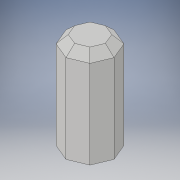
# Autodesk Inventor part: separator_battery
Saved by Autodesk Inventor 2019 (Build 230136000, 136)
## iProperties
Created: 2019-04-10
Part Number: separator_battery
Material: Generic
Document SubType Name: Modeling
Designer: jmc
Density: 1 g/cm^3
Appearance: Default
Author: jmc
Autodesk Inventor part; units mm, degrees
ref_plane "YZ Plane" through (0, 0, 0) normal (1, 0, 0) x (0, 1, 0)
ref_plane "XZ Plane" through (0, 0, 0) normal (0, 1, 0) x (-1, 0, 0)
ref_plane "XY Plane" through (0, 0, 0) normal (0, 0, 1) x (1, 0, 0)
sketch "Sketch1" plane through (0, 0, 0) normal (0, 1, 0) x (-1, 0, 0)
  circle A0 centre (0, 0) radius 1.5 construction
  line L0 (0, -1.5) -> (-1.0607, -1.0607)
  line L1 (-1.0607, -1.0607) -> (-1.5, 0)
  line L2 (-1.5, 0) -> (-1.0607, 1.0607)
  line L3 (-1.0607, 1.0607) -> (0, 1.5)
  line L4 (0, 1.5) -> (1.0607, 1.0607)
  line L5 (1.0607, 1.0607) -> (1.5, 0)
  line L6 (1.5, 0) -> (1.0607, -1.0607)
  line L7 (1.0607, -1.0607) -> (0, -1.5)
  dimension "d0" = 3
  constraints: 16 end point, 2 coincident, 1 vertical alignment, 19 other
extrude "Extrusion1" add sketch "Sketch1" along normal blind 6
chamfer "Chamfer1" distance 0.5 angle 45 8 edges at (0.5303, 6, 1.2803) (1.2803, 6, 0.5303) (1.2803, 6, -0.5303) (0.5303, 6, -1.2803) (-0.5303, 6, -1.2803) (-1.2803, 6, -0.5303) (-1.2803, 6, 0.5303) (-0.5303, 6, 1.2803)
body "Solid1"
